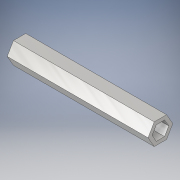
# Autodesk Inventor part: Metal Fastener
Saved by Autodesk Inventor 2018 (Build 220112000, 112)
## iProperties
Created: 2018-10-18
Part Number: Metal Fastener
Material: Generic
Document SubType Name: Modeling
Designer: USER
Density: 1 g/cm^3
Appearance: Machined - Aluminum
Author: USER
Autodesk Inventor part; units mm, degrees
ref_plane "YZ Plane" through (0, 0, 0) normal (1, 0, 0) x (0, 1, 0)
ref_plane "XZ Plane" through (0, 0, 0) normal (0, 1, 0) x (-1, 0, 0)
ref_plane "XY Plane" through (0, 0, 0) normal (0, 0, 1) x (1, 0, 0)
sketch "Sketch1" plane through (0, 0, 0) normal (1, 0, 0) x (0, 1, 0)
  line L0 (0, -1.4986) -> (-1.2978, -0.7493)
  line L1 (-1.2978, -0.7493) -> (-1.2978, 0.7493)
  line L2 (-1.2978, 0.7493) -> (0, 1.4986)
  line L3 (0, 1.4986) -> (1.2978, 0.7493)
  line L4 (1.2978, 0.7493) -> (1.2978, -0.7493)
  line L5 (1.2978, -0.7493) -> (0, -1.4986)
  line L6 (1.9295, -1.114) -> (1.9295, 1.114)
  line L7 (1.9295, 1.114) -> (0, 2.228)
  line L8 (0, 2.228) -> (-1.9295, 1.114)
  line L9 (-1.9295, 1.114) -> (-1.9295, -1.114)
  line L10 (-1.9295, -1.114) -> (0, -2.228)
  line L11 (0, -2.228) -> (1.9295, -1.114)
  point P0 (0, 0)
  point P1 (0, 0)
  dimension "d0" = 1.4986
  constraints: 24 end point, 1 coincident, 18 other
  measures "d0" distance of L0.start point (0, 0)
extrude "Extrusion1" add sketch "Sketch1" along normal blind 25.4
body "Solid1"
